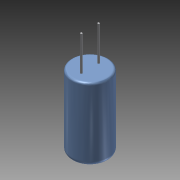
# Autodesk Inventor part: Capacitor
Saved by Autodesk Inventor 2014 (Build 180170000, 170)
## iProperties
Created: 2015-04-18
Part Number: Capacitor
Material: Generic
Document SubType Name: Modeling
Designer: Owner
Density: 1 g/cm^3
Appearance: Default
Author: Owner
Autodesk Inventor part; units mm, degrees
ref_plane "YZ Plane" through (0, 0, 0) normal (1, 0, 0) x (0, 1, 0)
ref_plane "XZ Plane" through (0, 0, 0) normal (0, 1, 0) x (-1, 0, 0)
ref_plane "XY Plane" through (0, 0, 0) normal (0, 0, 1) x (1, 0, 0)
sketch "Sketch1" plane through (0, 0, 0) normal (0, 1, 0) x (-1, 0, 0)
  circle A0 centre (0, 0) radius 8
  dimension "d0" = 16
  constraints: 1 centre point, 1 coincident
  measures "d0" diameter of A0
extrude "Extrusion1" add sketch "Sketch1" along normal blind 31.5
sketch "Sketch2" plane through (0, 31.5, 0) normal (0, 1, 0) x (1, 0, 0)
  circle A0 centre (0, 0) radius 8 projected
  circle A1 centre (0, 3.75) radius 0.4
  circle A2 centre (0, -3.75) radius 0.4
  dimension "d3" = 0.8
  dimension "d4" = 0.8
  dimension "d5" = 3.75
  dimension "d6" = 3.75
  constraints: 2 centre point
  measures "d3" diameter of A1
  measures "d4" diameter of A2
  measures "d5" distance of A0.centre A2.centre
  measures "d6" distance of A0.centre A1.centre
extrude "Extrusion2" add sketch "Sketch2" along normal blind 15 contours A1 | A2
fillet "Fillet1" radius 2 1 edges at (8, 0, 0)
fillet "Fillet2" radius 1 1 edges at (8, 31.5, 0)
body "Solid1"
